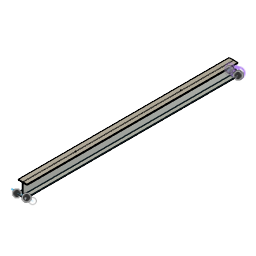
FEA (Autodesk Fusion 360 design; units mm, degrees)
Autodesk Fusion 360 part; units mm, degrees
sketch "Sketch1" plane through (0, 0, 0) normal (0, 0, 1) x (1, 0, 0)
  line L0 (-35, -70) -> (215, -70)
  line L1 (215, -70) -> (215, -50)
  line L2 (215, -50) -> (-35, -50)
  line L3 (-35, -50) -> (-35, -70)
  line L4 (80, -50) -> (100, -50)
  line L5 (100, -50) -> (100, 250)
  line L6 (100, 250) -> (80, 250)
  line L7 (80, 250) -> (80, -50)
  line L8 (-35, 250) -> (-35, 270)
  line L9 (215, 250) -> (215, 270)
  line L10 (215, 250) -> (-35, 250)
  line L11 (-35, 250) -> (-35, 270)
  line L12 (-35, 270) -> (215, 270)
  line L13 (215, 270) -> (215, 250)
  dimension "d1" = 250
  dimension "d2" = 20
  dimension "d3" = 20
  dimension "d4" = 300
  dimension "d5" = 20
  dimension "d6" = 115
  dimension "d7" = 115
  dimension "d8" = 115
  dimension "d9" = 115
  constraint horizontal L0
  constraint vertical L1
  constraint horizontal L2
  constraint vertical L3
  constraint horizontal L4
  constraint vertical L5
  constraint horizontal L6
  constraint vertical L7
  constraint coincident L2 L4.start
  constraint perpendicular L2 L8
  constraint perpendicular L2 L9
  constraint horizontal L10
  constraint vertical L11
  constraint horizontal L12
  constraint vertical L13
  measures "d1" distance of L0.start L0.end
  measures "d2" distance of L0.start L2.end
  measures "d3" distance of L4.start L4.end
  measures "d4" distance of L4.start L6.end
  measures "d5" distance of L9.start L9.end
  measures "d6" distance of L2.end L4.start
  measures "d7" distance of L1.end L4.end
  measures "d8" distance of L6.end L8.start
  measures "d9" distance of L5.end L9.start
extrude "Extrude1" add sketch "Sketch1" along normal blind 6000
sketch "Sketch2" plane through (0, 270, 0) normal (0, 1, 0) x (-1, 0, 0)
  line L0 (-215, 0) -> (35, 0)
  line L1 (35, 0) -> (35, 6000)
  line L2 (35, 6000) -> (-215, 6000)
  line L3 (-215, 6000) -> (-215, 0)
  circle A0 centre (-100, 4500) radius 12.5
  circle A1 centre (-100, 1500) radius 12.5
  dimension "d12" = 25
  dimension "d13" = 1500
  dimension "d14" = 25
  dimension "d15" = 1500
  measures "d12" diameter of A0
  measures "d13" distance of L2 A0.centre
  measures "d14" diameter of A1
  measures "d15" distance of L0 A1.centre
extrude "Extrude2" add sketch "Sketch2" along normal blind 1 contours A0
extrude "Extrude3" add 1 faces at (100.9272, 271, 4491.2435) along direction (0, 1, 0) blind 0.01
sketch "Sketch3" plane through (0, 270, 0) normal (0, 1, 0) x (-1, 0, 0)
  circle A0 centre (-100, 4500) radius 12.5
  line L0 (-215, 0) -> (35, 0)
  line L1 (35, 0) -> (35, 6000)
  line L2 (35, 6000) -> (-215, 6000)
  line L3 (-215, 6000) -> (-215, 0)
  circle A1 centre (-85.9982, 1500) radius 12.5
  dimension "d20" = 25
  dimension "d21" = 1500
  measures "d20" diameter of A1
  measures "d21" distance of L0 A1.centre
extrude "Extrude4" add sketch "Sketch3" along normal blind 0.01 contours A1
sketch "Sketch4" plane through (0, -70, 0) normal (0, -1, 0) x (1, 0, 0)
  line L0 (-35, 0) -> (215, 0)
  line L1 (215, 0) -> (215, 6000)
  line L2 (215, 6000) -> (-35, 6000)
  line L3 (-35, 6000) -> (-35, 0)
  line L4 (-35, 0) -> (215, 0)
  line L5 (215, 0) -> (215, -24.7751)
  line L6 (215, -24.7751) -> (-35, -24.7751)
  line L7 (-35, -24.7751) -> (-35, 0)
  line L8 (-35, 6000) -> (215, 6000)
  line L9 (215, 6000) -> (215, 6030.0887)
  line L10 (215, 6030.0887) -> (-35, 6030.0887)
  line L11 (-35, 6030.0887) -> (-35, 6000)
  constraint horizontal L4
  constraint vertical L5
  constraint horizontal L6
  constraint vertical L7
  constraint coincident L0.start L3.end
  constraint horizontal L8
  constraint vertical L9
  constraint horizontal L10
  constraint vertical L11
  constraint coincident L2.end L3.start
extrude "Extrude5" add sketch "Sketch4" against normal blind 20 contours L0 L4 L5 L6 L7
sketch "Sketch5" plane through (0, -70, 0) normal (0, -1, 0) x (1, 0, 0)
  line L0 (215, -24.7751) -> (215, 6000)
  line L1 (215, 6000) -> (-35, 6000)
  line L2 (-35, 6000) -> (-35, -24.7751)
  line L3 (-35, -24.7751) -> (215, -24.7751)
  line L4 (-35, 6000) -> (215, 6000)
  line L5 (215, 6000) -> (215, 6045.5256)
  line L6 (215, 6045.5256) -> (-35, 6045.5256)
  line L7 (-35, 6045.5256) -> (-35, 6000)
  constraint horizontal L4
  constraint vertical L5
  constraint horizontal L6
  constraint vertical L7
  constraint coincident L1.end L2.start
extrude "Extrude6" add sketch "Sketch5" against normal blind 20 contours L1 L4 L5 L6 L7
sketch "Sketch6" plane through (0, -50, 0) normal (0, 1, 0) x (-1, 0, 0)
  line L0 (-80, 6000) -> (-80, 0)
  line L1 (-80, 0) -> (-100, 0)
  line L2 (-100, 0) -> (-100, 6000)
  line L3 (-100, 6000) -> (-80, 6000)
  line L4 (35, -24.7751) -> (35, 6045.5256)
  line L5 (35, 6045.5256) -> (-215, 6045.5256)
  line L6 (-215, 6045.5256) -> (-215, -24.7751)
  line L7 (-215, -24.7751) -> (35, -24.7751)
  line L8 (35, 0) -> (44.2199, 0)
  line L9 (-215, 6009.7723) -> (200, 6009.7723)
  line L10 (200, 6009.7723) -> (-385.0295, 6009.7723)
  line L11 (-228.2182, 6046.4588) -> (-228.2182, 6009.7723)
  line L12 (25.7445, 6045.5256) -> (28.1278, 6009.7723)
  line L13 (-212.657, -24.7751) -> (-212.657, -35.5984)
  line L14 (44.2199, 0) -> (35, 0)
  line L15 (-215, 0) -> (-224.2, 0)
  line L16 (55.9142, -33.1803) -> (55.9142, 0)
  line L17 (55.9142, 0) -> (35, 0)
  constraint coincident L4 L8.start
  constraint perpendicular L4 L8
  constraint perpendicular L6 L14
  constraint coincident L6 L9.start
  constraint perpendicular L4 L9
  constraint perpendicular L4 L10
  constraint coincident L10 L11.end
  constraint perpendicular L10 L11
  constraint coincident L5 L12.start
  constraint coincident L9 L12.end
  constraint vertical L13
  constraint coincident L7 L13.start
  constraint coincident L6 L15.start
  constraint vertical L16
  constraint horizontal L17
sketch "Sketch7" plane through (0, 0, 0) normal (0, 1, 0) x (1, 0, 0)
  line L0 (215, 24.7751) -> (-35, 24.7751)
  point P0 (80, 0)
  dimension "d28" = 24.7751
  measures "d28" distance of P0 L0
sketch "Sketch8" plane through (0, -70, 0) normal (0, -1, 0) x (1, 0, 0)
  line L0 (215, -24.7751) -> (215, 6045.5256)
  line L1 (215, 6045.5256) -> (-35, 6045.5256)
  line L2 (-35, 6045.5256) -> (-35, -24.7751)
  line L3 (-35, -24.7751) -> (215, -24.7751)
  line L4 (-35, -24.7751) -> (-35, 0)
  line L5 (215, 0) -> (215, -24.7751)
  line L6 (-35, 0) -> (215, 0)
  constraint coincident L2.end L3.start
  constraint coincident L2 L4.end
  constraint coincident L0 L5.start
  constraint coincident L0.start L3.end
  constraint perpendicular L5 L6
extrude "Extrude7" add sketch "Sketch8" along normal blind 1 contours L0 L2 L3 L4 L5 L6
sketch "Sketch9" plane through (0, -70, 0) normal (0, -1, 0) x (1, 0, 0)
  line L0 (-35, 0) -> (215, 0)
  line L1 (215, 0) -> (215, 6045.5256)
  line L2 (215, 6045.5256) -> (-35, 6045.5256)
  line L3 (-35, 6045.5256) -> (-35, 0)
  line L4 (-35, 6045.5256) -> (-35, 5996.9144)
  line L5 (215, 5996.9144) -> (-35, 5996.9144)
  line L6 (215, 6045.5256) -> (215, 5996.9144)
  line L7 (215, 6045.5256) -> (-35, 6045.5256)
  constraint coincident L2.end L3.start
  constraint coincident L3 L4.end
  constraint coincident L1 L5.start
  constraint perpendicular L4 L5
  constraint coincident L1.end L2.start
extrude "Extrude8" cut sketch "Sketch9" against normal blind 1 contours L1 L2 L3 L4 L5 L6 L7
